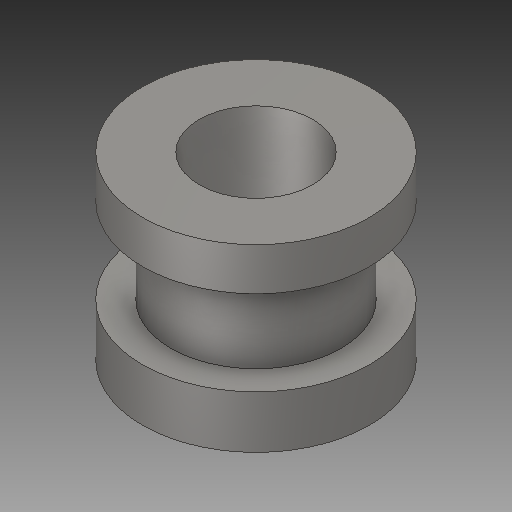
# Autodesk Inventor part: Groove_Mount_Adaptor_1_75mm
Saved by Autodesk Inventor 2019 (Build 230136000, 136)
## iProperties
Created: 2018-09-16
Part Number: Groove_Mount_Adaptor_1_75mm
Material: Generic
Document SubType Name: Modeling
Designer: Ax
Density: 1 g/cm^3
Appearance: Stainless - Brushed
Mass: 1.56713 g
Surface Area: 13.5447 cm^2
Volume: 1.56713 cm^3
Author: Ax
Autodesk Inventor part; units mm, degrees
ref_plane "YZ Plane" through (0, 0, 0) normal (1, 0, 0) x (0, 1, 0)
ref_plane "XZ Plane" through (0, 0, 0) normal (0, 1, 0) x (-1, 0, 0)
ref_plane "XY Plane" through (0, 0, 0) normal (0, 0, 1) x (1, 0, 0)
sketch "Sketch1" plane through (0, 0, 0) normal (0, 0, 1) x (1, 0, 0)
  line L0 (-2.1, -6.7) -> (-8, -6.7)
  line L1 (-8, -6.7) -> (-8, -3)
  line L2 (-8, -3) -> (-6, -3)
  line L3 (-6, -3) -> (-6, 3)
  line L4 (-6, 3) -> (-8, 3)
  line L5 (-8, 3) -> (-8, 6)
  line L6 (-8, 6) -> (-4, 6)
  line L7 (0, 0) -> (-16, 0) construction
  line L8 (0, -9.24) -> (0, 8.54) projected
  line L9 (-2.1, -6.7) -> (-2.1, -2.7)
  line L10 (-2.1, -2.7) -> (-4, -1)
  line L11 (-4, -1) -> (-4, 6)
  dimension "d1" = 8
  dimension "d2" = 3.7
  dimension "d3" = 3
  dimension "d4" = 6
  dimension "d5" = 6
  dimension "d7" = 4
  dimension "d8" = 2.1
  dimension "d9" = 7
  dimension "d11" = 4
  constraints: 22 end point, 4 perpendicular, 3 horizontal, 2 parallel, 1 symmetric about line, 1 vertical
  measures "d1" horizontal distance of L5.end L7.start
  measures "d2" distance of L0.end L1.end
  measures "d3" distance of L4.end L5.end
  measures "d4" horizontal distance of L7.start L2.end
  measures "d5" distance of L2.end L3.end
  measures "d7" horizontal distance of L7.start L6.end
  measures "d8" horizontal distance of L7.start L0.start
  measures "d9" distance of L10.end L6.end
  measures "d11" distance of L0.start L9.end
revolve "Revolution2" add sketch "Sketch1" angle 360 about axis through (0, -10, 0) along (0, 1, 0)
body "Solid2"
